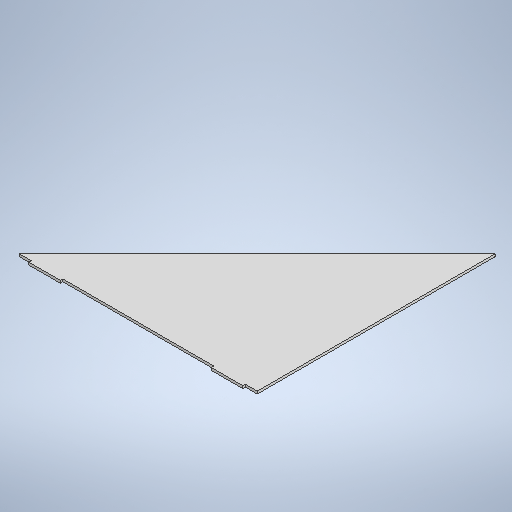
# Autodesk Inventor part: Trebuchet V1 - Truss Support
Saved by Autodesk Inventor 2025.2 (Build 292293000, 293)
## iProperties
Created: 2025-04-07
Part Number: Trebuchet V1 - Truss Support
Material: Generic
Document SubType Name: Modeling
Designer: Dylan
Density: 1 g/cm^3
Appearance: Default
Author: VRK99-0110
Title: Trebuchet - Truss Support
Subject: Trebuchet Project
Autodesk Inventor part; units mm, degrees
ref_plane "YZ Plane" through (0, 0, 0) normal (1, 0, 0) x (0, 1, 0)
ref_plane "XZ Plane" through (0, 0, 0) normal (0, 1, 0) x (-1, 0, 0)
ref_plane "XY Plane" through (0, 0, 0) normal (0, 0, 1) x (1, 0, 0)
sketch "Sketch1" plane through (0, 0, 0) normal (0, 1, 0) x (-1, 0, 0)
  line L0 (0, 0) -> (301.4, 0)
  line L1 (301.4, 0) -> (42.4, -259)
  line L2 (42.4, -259) -> (0, -301.4)
  line L3 (0, -301.4) -> (0, 0)
  line L4 (301.4, 0) -> (286.4, 0)
  line L5 (286.4, 0) -> (286.4, 3.2)
  line L6 (286.4, 3.2) -> (246.4, 3.2)
  line L7 (246.4, 3.2) -> (246.4, 0)
  line L8 (0, 0) -> (15, 0)
  line L9 (15, 0) -> (15, 3.2)
  line L10 (15, 3.2) -> (55, 3.2)
  line L11 (55, 3.2) -> (55, 0)
  line L12 (55, 0) -> (15, 0)
  dimension "d0" = 301.4
  dimension "d1" = 45
  dimension "d2" = 15
  dimension "d3" = 3.2
  dimension "d4" = 40
  dimension "d5" = 15
  dimension "d6" = 40
  constraints: 26 end point, 7 perpendicular, 5 point on line, 1 collinear, 1 horizontal
  measures "d0" distance of L0.start L0.end
  measures "d1" angle of L0 L1
  measures "d2" distance of L0.end L4.end
  measures "d3" distance of L4.end L5.end
  measures "d4" distance of L5.end L6.end
  measures "d5" distance of L0.start L8.end
  measures "d6" distance of L9.end L10.end
extrude "Extrusion1" add sketch "Sketch1" along normal blind 3.175
body "Solid1"
